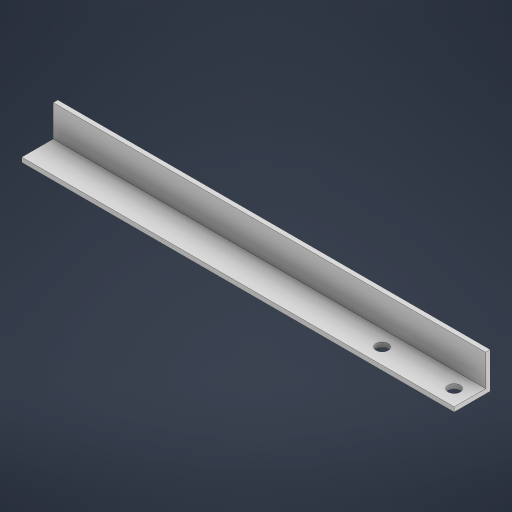
# Autodesk Inventor part: wing
Saved by Autodesk Inventor 2024 (Build 280153000, 153)
## iProperties
Created: 2023-12-24
Part Number: wing
Material: Generic
Document SubType Name: Modeling
Designer: elite
Density: 1 g/cm^3
Appearance: Default
Author: elite
Autodesk Inventor part; units mm, degrees
ref_plane "YZ Plane" through (0, 0, 0) normal (1, 0, 0) x (0, 1, 0)
ref_plane "XZ Plane" through (0, 0, 0) normal (0, 1, 0) x (-1, 0, 0)
ref_plane "XY Plane" through (0, 0, 0) normal (0, 0, 1) x (1, 0, 0)
sketch "Sketch1" plane through (0, 0, 0) normal (1, 0, 0) x (0, 1, 0)
  line L0 (0, 0) -> (1.6002, 0)
  line L1 (1.6002, 0) -> (1.6002, -12.7)
  line L2 (1.6002, -12.7) -> (0, -12.7)
  line L3 (0, -12.7) -> (0, 0)
  line L4 (0, -12.7) -> (0, -11.0998)
  line L5 (0, -11.0998) -> (12.7, -11.0998)
  line L6 (12.7, -11.0998) -> (12.7, -12.7)
  line L7 (12.7, -12.7) -> (0, -12.7)
  line L8 (0, -12.7) -> (0, -11.0998)
  point P0 (1.6002, -11.0998)
  dimension "d0" = 1.6002
  dimension "d1" = 12.7
  dimension "d2" = 1.6002
  dimension "d3" = 12.7
  constraints: 18 end point, 4 parallel, 2 horizontal, 2 perpendicular, 2 point on line
  measures "d0" distance of L1.end L2.end
  measures "d1" distance of L2.end L0.start
  measures "d2" distance of L2.end L4.end
  measures "d3" distance of L6.end L7.end
extrude "Extrusion1" add sketch "Sketch1" along normal blind 152.4
sketch "Sketch2" plane through (0, 1.6002, 0) normal (0, 1, 0) x (1, 0, 0)
  line L0 (0, 0) -> (152.4, 0) projected
  line L1 (0, 11.0998) -> (152.4, 11.0998) projected
  line L2 (152.4, 0) -> (141.3002, 0)
  line L3 (141.3002, 0) -> (141.3002, 11.0998)
  line L4 (141.3002, 11.0998) -> (152.4, 11.0998)
  line L5 (152.4, 11.0998) -> (152.4, 0)
  line L6 (152.4, 0) -> (141.3002, 11.0998)
  circle A0 centre (146.8501, 5.5499) radius 2.1082
  line L7 (146.8501, 5.5499) -> (121.4501, 5.5499)
  circle A1 centre (121.4501, 5.5499) radius 2.1082
  dimension "d6" = 11.0998
  dimension "d7" = 4.2164
  dimension "d8" = 25.4
  constraints: 12 end point, 2 centre point, 2 horizontal, 2 parallel, 1 coincident, 1 midpoint, 1 perpendicular, 1 point on line
  measures "d6" distance of L3.end L4.end
  measures "d7" diameter of A0
  measures "d8" distance of L7.start L7.end
extrude "Extrusion2" cut sketch "Sketch2" against normal blind 152.4 contours A0 L7 L6 | L6 A0 | A0 L6 L7 | A1
body "Solid1"
